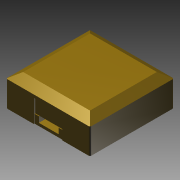
# Autodesk Inventor part: UB216SKG035D-NR
Saved by Autodesk Inventor 2015 SP1 (Build 190203100, 203)
## iProperties
Category: Electrical
Company: Autodesk Inc.
Created: 2014-12-16
Part Number: UB216SKG035D-NR
Catalog Web Link: http://www.nkkswitches.com/
Description: AT3073, AT3077-Non-Illuminated Pushbuttons - Series UB2
Vendor: NKK Switches
Document SubType Name: Modeling
Designer: Autodesk Inc.
Manufacturer: NKKSWITCHES
Mass: 1.20723 g
Surface Area: 7.52236 cm^2
Volume: 1.20723 cm^3
Density: 1 g/cm^3
Material: Generic
Appearance: PSOLRGB-255-191-0
Title: UB2-5Dni_cap
Author: Autodesk Inc.
Comments: Non-Illuminated Pushbuttons - Series UB2
Autodesk Inventor part; units mm, degrees
sketch "Sketch_13" plane through (0, 0, 0) normal (0, 0, 1) x (1, 0, 0)
  line L0 (-7.5057, 0) -> (7.5057, 0)
  line L1 (7.5057, 0) -> (7.5057, 5.588)
  line L2 (7.5057, 5.588) -> (-7.5057, 5.588)
  line L3 (-7.5057, 5.588) -> (-7.5057, 0)
  constraints: 8 end point
extrude "Extrusion1" add sketch "Sketch_13" along normal mid plane 15.0114
sketch "Sketch_21" plane through (0, 0, 0) normal (0, 1, 0) x (-1, 0, 0)
  line L0 (8.89, 8.89) -> (-8.89, 8.89)
  line L1 (-8.89, 8.89) -> (-8.89, -8.89)
  line L2 (-8.89, -8.89) -> (8.89, -8.89)
  line L3 (8.89, -8.89) -> (8.89, 8.89)
  line L4 (7.5057, -7.2517) -> (7.5057, 7.2517)
  arc A0 (7.5057, 7.2517) -> (7.2517, 7.5057) centre (7.2517, 7.2517) ccw
  line L5 (7.2517, 7.5057) -> (-7.2517, 7.5057)
  arc A1 (-7.2517, 7.5057) -> (-7.5057, 7.2517) centre (-7.2517, 7.2517) ccw
  line L6 (-7.5057, 7.2517) -> (-7.5057, -7.2517)
  arc A2 (-7.5057, -7.2517) -> (-7.2517, -7.5057) centre (-7.2517, -7.2517) ccw
  line L7 (-7.2517, -7.5057) -> (7.2517, -7.5057)
  arc A3 (7.2517, -7.5057) -> (7.5057, -7.2517) centre (7.2517, -7.2517) ccw
  constraints: 16 end point, 8 point on circle, 4 centre point
extrude "Extrusion2" cut sketch "Sketch_21" along normal blind 7.62
sketch "Sketch_14" plane through (0, 0, 0) normal (0, 0, 1) x (1, 0, 0)
  line L0 (-7.5057, 8.128) -> (-7.5057, 4.572)
  line L1 (-7.5057, 4.572) -> (-3.6957, 7.112)
  line L2 (-3.6957, 7.112) -> (3.6957, 7.112)
  line L3 (3.6957, 7.112) -> (7.5057, 4.572)
  line L4 (7.5057, 4.572) -> (7.5057, 8.128)
  line L5 (7.5057, 8.128) -> (-7.5057, 8.128)
  constraints: 12 end point
extrude "Extrusion3" cut sketch "Sketch_14" along normal mid plane 15.24
sketch "Sketch_15" plane through (0, 0, 0) normal (1, 0, 0) x (0, 1, 0)
  line L0 (8.128, 7.5057) -> (4.572, 7.5057)
  line L1 (4.572, 7.5057) -> (7.112, 3.6957)
  line L2 (7.112, 3.6957) -> (7.112, -3.6957)
  line L3 (7.112, -3.6957) -> (4.572, -7.5057)
  line L4 (4.572, -7.5057) -> (8.128, -7.5057)
  line L5 (8.128, -7.5057) -> (8.128, 7.5057)
  constraints: 12 end point
extrude "Extrusion4" cut sketch "Sketch_15" along normal mid plane 15.24
sketch "Sketch_17" plane through (0, 0, 7.5057) normal (0, 0, 1) x (1, 0, 0)
  line L0 (-2.54, 0) -> (2.54, 0)
  line L1 (2.54, 0) -> (2.54, 4.064)
  line L2 (2.54, 4.064) -> (-2.54, 4.064)
  line L3 (-2.54, 4.064) -> (-2.54, 0)
  constraints: 8 end point
extrude "Extrusion5" cut sketch "Sketch_17" against normal blind 0.127
sketch "Sketch_18" plane through (0, 0, 7.5057) normal (0, 0, 1) x (1, 0, 0)
  line L0 (-2.54, 1.524) -> (2.54, 1.524)
  line L1 (2.54, 1.524) -> (2.54, 4.064)
  line L2 (2.54, 4.064) -> (-2.54, 4.064)
  line L3 (-2.54, 4.064) -> (-2.54, 1.524)
  constraints: 8 end point
extrude "Extrusion6" cut sketch "Sketch_18" against normal blind 0.254
sketch "Sketch_19" plane through (0, 0, 7.5057) normal (0, 0, 1) x (1, 0, 0)
  line L0 (-1.778, 0.508) -> (1.778, 0.508)
  line L1 (1.778, 0.508) -> (1.778, 1.524)
  line L2 (1.778, 1.524) -> (-1.778, 1.524)
  line L3 (-1.778, 1.524) -> (-1.778, 0.508)
  constraints: 8 end point
extrude "Extrusion7" cut sketch "Sketch_19" against normal blind 1.27
ref_plane "lens_to_body_XY" through (0, 0, 0) normal (0, 1, 0) x (1, 0, 0)
ref_plane "lens_to_body_YZ" through (0, 0, 0) normal (1, 0, 0) x (0, 0, -1)
ref_plane "lens_to_body_ZX" through (0, 0, 0) normal (0, 0, -1) x (0, 1, 0)
body "Solid1"
